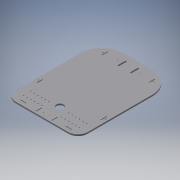
# Autodesk Inventor part: Base
Saved by Autodesk Inventor 2018 (Build 220112000, 112)
## iProperties
Created: 2018-05-02
Part Number: Base
Material: Generic
Document SubType Name: Modeling
Designer: Ajith Thomas
Density: 1 g/cm^3
Appearance: Default
Author: Ajith Thomas
Autodesk Inventor part; units mm, degrees
ref_plane "YZ Plane" through (0, 0, 0) normal (1, 0, 0) x (0, 1, 0)
ref_plane "XZ Plane" through (0, 0, 0) normal (0, 1, 0) x (-1, 0, 0)
ref_plane "XY Plane" through (0, 0, 0) normal (0, 0, 1) x (1, 0, 0)
sketch "Sketch1" plane through (0, 0, 0) normal (0, 1, 0) x (-1, 0, 0)
  line L0 (150, 200) -> (-150, 200)
  line L1 (-150, 200) -> (-150, -200)
  line L2 (-150, -200) -> (150, -200)
  line L3 (150, -200) -> (150, 200)
  line L4 (150, 200) -> (-150, -200) construction
  line L5 (-150, 200) -> (150, -200) construction
  point P0 (0, 0)
  dimension "d0" = 300
  dimension "d1" = 400
  constraints: 12 end point, 2 midpoint, 2 parallel, 1 horizontal, 1 perpendicular
  measures "d0" distance of L2.end L1.end
  measures "d1" distance of L1.end L0.end
extrude "Extrusion1" add sketch "Sketch1" along normal blind 6
sketch "Sketch2" plane through (0, 6, 0) normal (0, 1, 0) x (1, 0, 0)
  line L0 (116.2, -158) -> (86.2, -158) construction
  line L1 (86.2, -162) -> (116.2, -162) construction
  arc A0 (86.2, -158) -> (86.2, -162) centre (86.2, -160) ccw construction
  arc A1 (116.2, -162) -> (116.2, -158) centre (116.2, -160) ccw construction
  line L2 (86.2, -132) -> (116.2, -132) construction
  line L3 (116.2, -128) -> (86.2, -128) construction
  arc A2 (116.2, -132) -> (116.2, -128) centre (116.2, -130) ccw construction
  arc A3 (86.2, -128) -> (86.2, -132) centre (86.2, -130) ccw construction
  line L4 (-116.2, -162) -> (-86.2, -162) construction
  line L5 (-86.2, -158) -> (-116.2, -158) construction
  arc A4 (-116.2, -158) -> (-116.2, -162) centre (-116.2, -160) ccw construction
  arc A5 (-86.2, -162) -> (-86.2, -158) centre (-86.2, -160) ccw construction
  arc A6 (-86.2, -132) -> (-86.2, -128) centre (-86.2, -130) ccw construction
  line L6 (-86.2, -128) -> (-116.2, -128) construction
  line L7 (-116.2, -132) -> (-86.2, -132) construction
  arc A7 (-116.2, -128) -> (-116.2, -132) centre (-116.2, -130) ccw construction
  line L8 (-116.2, -162) -> (-86.2, -162) construction
  line L9 (-86.2, -158) -> (-116.2, -158) construction
  circle A8 centre (-116.2, -160) radius 2
  circle A9 centre (-116.2, -130) radius 2
  circle A10 centre (-86.2, -130) radius 2
  circle A11 centre (-101.2, -130) radius 2
  circle A12 centre (-101.2, -160) radius 2
  circle A13 centre (-86.2, -160) radius 2
  circle A14 centre (86.2, -160) radius 2
  circle A15 centre (116.2, -160) radius 2
  circle A16 centre (101.2, -160) radius 2
  circle A17 centre (101.2, -130) radius 2
  circle A18 centre (86.2, -130) radius 2
  circle A19 centre (116.2, -130) radius 2
  circle A20 centre (-71.2, -160) radius 2
  circle A21 centre (-71.2, -130) radius 2
  circle A22 centre (-56.2, -160) radius 2
  circle A23 centre (-56.2, -130) radius 2
  circle A24 centre (-41.2, -160) radius 2
  circle A25 centre (-41.2, -130) radius 2
  circle A26 centre (71.2, -130) radius 2
  circle A27 centre (71.2, -160) radius 2
  circle A28 centre (56.2, -130) radius 2
  circle A29 centre (56.2, -160) radius 2
  circle A30 centre (41.2, -130) radius 2
  circle A31 centre (41.2, -160) radius 2
  point P0 (0, 0)
  point P1 (-71.2, -158)
  point P2 (-56.2, -158)
  point P3 (-41.2, -158)
  dimension "d4" = 15
  dimension "d5" = 15
  dimension "d6" = 15
  dimension "d7" = 15
  dimension "d17" = 15
  dimension "d24" = 15
  dimension "d29" = 15
  constraints: 17 centre point, 8 coincident, 7 vertical alignment, 5 horizontal, 4 tangent, 1 concentric, 38 other
  measures "d4" distance of A6.centre A11.centre
  measures "d5" distance of A5.centre A12.centre
  measures "d6" distance of A1.centre A16.centre
  measures "d7" distance of A2.centre A17.centre
  measures "d17" distance of point (-86.2, -160) point (-71.2, -160)
  measures "d24" distance of A18.centre A26.centre
  measures "d29" distance of A29.centre A31.centre
extrude "Extrusion2" cut sketch "Sketch2" against normal blind 10
sketch "Sketch4" plane through (0, 6, 0) normal (0, 1, 0) x (1, 0, 0)
  circle A0 centre (0, -125) radius 15
  line L0 (-150, -200) -> (150, -200) projected
  line L1 (-150, 200) -> (-150, -200) projected
  point P0 (0, 0)
  dimension "d30" = 30
  dimension "d31" = 75
  dimension "d32" = 150
  constraints: 1 centre point
  measures "d30" diameter of A0
  measures "d31" distance from line of L0 A0.centre
  measures "d32" distance from line of L1 A0.centre
extrude "Extrusion4" cut sketch "Sketch4" against normal blind 10
sketch "Sketch5" plane through (0, 6, 0) normal (0, 1, 0) x (1, 0, 0)
  line L0 (28.9, 177) -> (28.9, 143) projected
  line L1 (22.9, 143) -> (22.9, 177) projected
  line L2 (28.9, 177) -> (22.9, 177) projected
  line L3 (28.9, 143) -> (22.9, 143) projected
  line L4 (-22.9, 177) -> (-22.9, 143) projected
  line L5 (-28.9, 143) -> (-28.9, 177) projected
  line L6 (-28.9, 177) -> (-22.9, 177) projected
  line L7 (-28.9, 143) -> (-22.9, 143) projected
  point P0 (0, 0)
extrude "Extrusion5" cut sketch "Sketch5" against normal blind 10
sketch "Sketch6" plane through (0, 6, 0) normal (0, 1, 0) x (1, 0, 0)
  circle A0 centre (45, 160) radius 1.5 projected
  circle A1 centre (-45, 160) radius 1.5 projected
  point P0 (0, 0)
extrude "Extrusion6" cut sketch "Sketch6" against normal blind 10
fillet "Fillet1" radius 40 2 edges at (-150, 3, 200) (150, 3, 200)
fillet "Fillet2" radius 90 2 edges at (150, 3, -200) (-150, 3, -200)
sketch "Sketch7" plane through (0, 6, 0) normal (0, 1, 0) x (1, 0, 0)
  line L0 (-34.75, -192) -> (-34.75, -168) projected
  line L1 (-34.75, -168) -> (-31.75, -168) projected
  line L2 (-31.75, -192) -> (-31.75, -168) projected
  line L3 (-34.75, -192) -> (-31.75, -192) projected
  line L4 (31.75, -192) -> (31.75, -168) projected
  line L5 (31.75, -168) -> (34.75, -168) projected
  line L6 (34.75, -192) -> (34.75, -168) projected
  line L7 (31.75, -192) -> (34.75, -192) projected
  point P0 (0, 0)
extrude "Extrusion7" cut sketch "Sketch7" against normal blind 10
sketch "Sketch8" plane through (0, 6, 0) normal (0, 1, 0) x (1, 0, 0)
  circle A0 centre (12.5, -180) radius 1.5 projected
  circle A1 centre (0, -192.5) radius 1.5 projected
  circle A2 centre (-12.5, -180) radius 1.5 projected
  point P0 (0, 0)
extrude "Extrusion8" cut sketch "Sketch8" against normal blind 10
sketch "Sketch9" plane through (0, 6, 0) normal (0, 1, 0) x (1, 0, 0)
  line L0 (-110, -200) -> (110, -200) projected
  line L1 (150, -160) -> (150, 110) projected
  line L2 (-150, 110) -> (-150, -160) projected
  line L3 (60, 200) -> (-60, 200) projected
  line L4 (0, -200) -> (0, 200) construction
  line L5 (60, 200) -> (-60, 200) construction
  line L6 (83, -185) -> (107, -185) projected
  line L7 (83, -185) -> (83, -182) projected
  line L8 (107, -182) -> (83, -182) projected
  line L9 (107, -185) -> (107, -182) projected
  line L10 (132, -63) -> (132, -87) projected
  line L11 (132, -63) -> (135, -63) projected
  line L12 (135, -87) -> (135, -63) projected
  line L13 (132, -87) -> (135, -87) projected
  line L14 (97, 172) -> (97, 148) projected
  line L15 (97, 172) -> (100, 172) projected
  line L16 (100, 148) -> (100, 172) projected
  line L17 (97, 148) -> (100, 148) projected
  line L18 (-83, -185) -> (-107, -185)
  line L19 (-83, -185) -> (-83, -182)
  line L20 (-107, -182) -> (-83, -182)
  line L21 (-107, -185) -> (-107, -182)
  line L22 (-132, -63) -> (-132, -87)
  line L23 (-132, -63) -> (-135, -63)
  line L24 (-135, -87) -> (-135, -63)
  line L25 (-132, -87) -> (-135, -87)
  line L26 (-97, 172) -> (-97, 148)
  line L27 (-97, 172) -> (-100, 172)
  line L28 (-100, 148) -> (-100, 172)
  line L29 (-97, 148) -> (-100, 148)
  point P0 (0, 0)
  constraints: 26 end point, 12 symmetric about line, 2 midpoint
extrude "Extrusion9" cut sketch "Sketch9" against normal blind 10
sketch "Sketch10" plane through (0, 6, 0) normal (0, 1, 0) x (1, 0, 0)
  line L0 (135, -63) -> (135, -87) construction
  line L1 (100, 172) -> (100, 148) construction
  circle A0 centre (140.5, -75) radius 4.5 construction
  circle A1 centre (140.5, -75) radius 2
  circle A2 centre (105.5, 160) radius 4.5 construction
  circle A3 centre (105.5, 160) radius 2
  line L2 (-110, -200) -> (110, -200) projected
  line L3 (60, 200) -> (-60, 200) projected
  line L4 (0, -200) -> (0, 200) construction
  circle A4 centre (-140.5, -75) radius 4.5 construction
  circle A5 centre (-140.5, -75) radius 2
  circle A6 centre (-105.5, 160) radius 4.5 construction
  circle A7 centre (-105.5, 160) radius 2
  point P0 (0, 0)
  dimension "d47" = 9
  dimension "d48" = 12
  dimension "d50" = 5.5
  dimension "d51" = 4
  dimension "d52" = 9
  dimension "d53" = 12
  dimension "d54" = 5.5
  dimension "d55" = 4
  constraints: 8 centre point, 4 coincident, 4 symmetric about line, 2 end point, 2 midpoint, 4 other
  measures "d47" diameter of A0
  measures "d48" vertical distance of L0.end A0.centre
  measures "d50" distance from line of L0 A0.centre
  measures "d51" diameter of A1
  measures "d52" diameter of A2
  measures "d53" vertical distance of L1.end A2.centre
  measures "d54" distance from line of L1 A2.centre
  measures "d55" diameter of A3
extrude "Extrusion10" cut sketch "Sketch10" against normal blind 10
body "Solid1"
